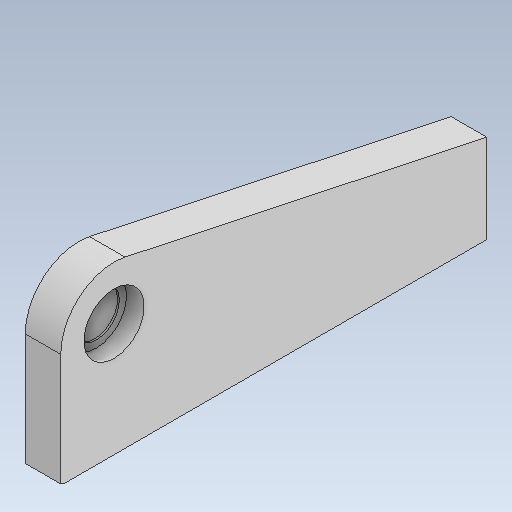
# Autodesk Inventor part: Waffenhalterung rechts 70mm
Saved by Autodesk Inventor 2026.4 (Build 304435030, 435C)
## iProperties
Created: 2026-11-24
Part Number: Waffenhalterung rechts 70mm
Material: Generisch
Document SubType Name: Modeling
Designer: weira
Density: 1 g/cm^3
Appearance: Vorgabe
Author: weira
Autodesk Inventor part; units mm, degrees
ref_plane "YZ Plane" through (0, 0, 0) normal (1, 0, 0) x (0, 1, 0)
ref_plane "XZ Plane" through (0, 0, 0) normal (0, 1, 0) x (-1, 0, 0)
ref_plane "XY Plane" through (0, 0, 0) normal (0, 0, 1) x (1, 0, 0)
sketch "Skizze1" plane through (0, 0, 0) normal (1, 0, 0) x (0, 1, 0)
  line L0 (0, 0) -> (100, 0)
  line L1 (100, 0) -> (100, 25)
  line L2 (100, 25) -> (0, 25)
  line L3 (0, 25) -> (0, 0)
  circle A0 centre (-5, 32) radius 8.5
  circle A1 centre (-5, 32) radius 15
  line L4 (100, 25) -> (-1.879, 46.6717)
  line L5 (0, 0) -> (-17.0625, 23.084)
  circle A2 centre (-5, 32) radius 35
  line L6 (-5, 32) -> (52.8273, 16)
  circle A3 centre (52.8273, 16) radius 16
  line L7 (-20, 32) -> (-20, -9.1489)
  line L8 (0, 0) -> (-36.2832, 0)
  point P0 (28.7326, 22.6667)
  point P1 (37.4067, 20.2667)
  point P2 (-19.1774, 0)
  point P3 (-20, 0.3772)
  dimension "d6" = 70
  dimension "d7" = 32
  dimension "d1" = 100
  dimension "d2" = 17
  dimension "d3" = 5
  dimension "d4" = 30
  dimension "d5" = 32
  dimension "d8" = 60
  dimension "d9" = 9
  constraints: 18 end point, 4 coincident, 3 horizontal, 3 point on circle, 3 tangent, 2 centre point, 2 parallel, 2 point on line, 1 perpendicular, 1 vertical, 6 other
  measures "d1" distance of L1.end L2.end
  measures "d2" diameter of A0
  measures "d3" distance from line of L3 A0.centre
  measures "d4" diameter of A1
  measures "d5" distance from line of L0 A0.centre
  measures "d8" distance of L6.start L6.end
  measures "d9" distance of point (37.407, 20.267) point (28.733, 22.667)
extrude "Extrusion1" add sketch "Skizze1" along normal blind 10 contours L3 A1 L2 L6 A2 L0 | L5 A1 L3 | L8 A2 L7 A1 L5 | A2 L6 A3 L0 | A1 L2 L3 | L3 L2 A1 | A3 L2 L1 L0 | A3 L2 | L6 L2 A2 | A2 L2 A3 L6 | A1 L6 L2 | A2 L4 L2 A3 | L2 L6 A1 L4 A2 | A3 L2 | A0
sketch "Skizze2" plane through (10, 0, 0) normal (1, 0, 0) x (0, 0, -1)
  line L0 (0, -19.1774) -> (0, 100) projected
  line L1 (0, 100) -> (-25, 100) projected
  line L2 (-25, 100) -> (-46.6717, -1.879) projected
  arc A0 (-46.6717, -1.879) -> (-32, -20) centre (-32, -5) ccw projected
  line L3 (-32, -20) -> (-0.3772, -20) projected
  arc A1 (-0.3772, -20) -> (0, -19.1774) centre (-32, -5) ccw projected
  circle A2 centre (-32, -5) radius 8.5
  circle A3 centre (-32, -5) radius 6.5
  point P0 (0, 0)
  dimension "d12" = 17
  dimension "d13" = 13
  constraints: 2 centre point, 2 coincident
  measures "d12" diameter of A2
  measures "d13" diameter of A3
extrude "Extrusion2" cut sketch "Skizze2" against normal blind 5 contours A2
extrude "Extrusion3" cut sketch "Skizze2" against normal blind 5.5 contours A3
